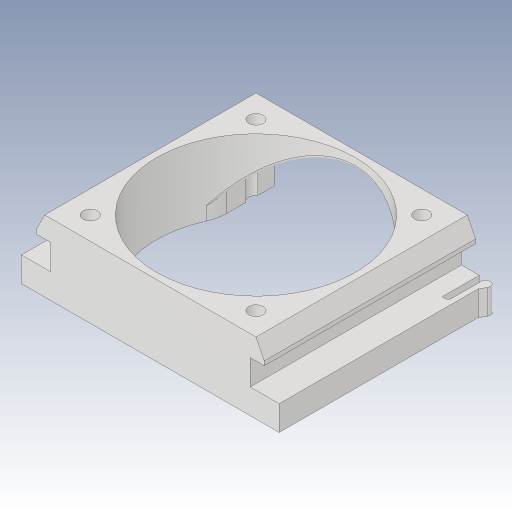
# Autodesk Inventor part: BT016_huenin20_24
Saved by Autodesk Inventor 2023.3 (Build 273359000, 359)
## iProperties
Company: HTBLA Kaindorf
RuleStatus: InUse
Created: 2025-01-29
Part Number: BT016_huenin20_24
Project: Fiberprinter-Hotend
Material: ABS-Kunststoff
Description: Bauteilkühllüfter_befestigung
Document SubType Name: Modeling
Designer: huenin20
Density: 1.06 g/cm^3
Appearance: Glatt - Weiß
Mass: 1.79395 g
Surface Area: 23.0026 cm^2
Volume: 1.69241 cm^3
AfterDocNew0: iProperties-Editor_aufrufen
Author: nicob
Keywords: 2024
Autodesk Inventor part; units mm, degrees
ref_plane "YZ Plane" through (0, 0, 0) normal (1, 0, 0) x (0, 1, 0)
ref_plane "XZ Plane" through (0, 0, 0) normal (0, 1, 0) x (-1, 0, 0)
ref_plane "XY Plane" through (0, 0, 0) normal (0, 0, 1) x (1, 0, 0)
sketch "Skizze3" plane through (0, 0, 0) normal (1, 0, 0) x (0, 1, 0)
  line L0 (0, 0) -> (24.1, 0)
  line L1 (24.1, 0) -> (24.1, -3.075)
  line L2 (24.1, -3.075) -> (27.6, -3.075)
  line L3 (27.6, -3.075) -> (27.6, -6.075)
  line L4 (27.6, -6.075) -> (-3.5, -6.075)
  line L5 (-3.5, -6.075) -> (-3.5, -3.075)
  line L6 (-3.5, -3.075) -> (0, -3.075)
  line L7 (0, -3.075) -> (0, 0)
  line L8 (0, 0) -> (-1.7, 0)
  line L9 (-1.7, 0) -> (-1.7, 2.5)
  line L10 (-1.7, 2.5) -> (25.8, 2.5)
  line L11 (25.8, 2.5) -> (25.8, 0)
  line L12 (25.8, 0) -> (24.1, 0)
  dimension "d4" = 24.1
  dimension "d5" = 3.075
  dimension "d6" = 3
  dimension "d7" = 3.5
  dimension "d15" = 27.5
  dimension "d16" = 2.5
  constraints: 26 end point, 9 perpendicular, 3 collinear, 3 point on line, 2 horizontal, 1 horizontal alignment
  measures "d4" distance of L0.start L0.end
  measures "d5" distance of L0.end L1.end
  measures "d6" distance of L2.end L3.end
  measures "d7" distance of L5.end L6.end
  measures "d15" distance of L9.end L10.end
  measures "d16" distance of L8.end L9.end
extrude "Extrusion3" add sketch "Skizze3" along normal blind 25.5
ref_plane "Arbeitsebene1" through (0, 12.05, -3.075) normal (0, 1, 0) x (1, 0, 0)
sketch "Skizze4" plane through (0, 12.05, -3.075) normal (0, 1, 0) x (1, 0, 0)
  line L0 (0, 3) -> (0, 0) projected
  line L1 (0, 3) -> (25.5, 3) projected
  line L2 (0, -4.5) -> (8.9382, 3)
  line L3 (0, 0) -> (0, -3.075) projected
  line L4 (0, -3.075) -> (0, -5.575) projected
  dimension "d10" = 7.5
  dimension "d14" = 140
  constraints: 2 end point, 2 point on line
  measures "d10" distance of L0.start L2.start
  measures "d14" angle of L1 L2
extrude "Extrusion4" cut sketch "Skizze4" along normal mid plane 21
chamfer "Fase1" distance 1 distance2 2 2 edges at (12.75, -1.7, 2.5) (12.75, 25.8, 2.5) measured on face at (12.75, 25.3, 2.5) measured on face at (12.75, -1.2, 2.5)
sketch "Skizze5" plane through (0, -0.7, 2.5) normal (0, 0, 1) x (1, 0, 0)
  circle A0 centre (12.75, 12.75) radius 12
  line L0 (25.5, 25.5) -> (25.5, 0) projected
  point P0 (0, 0.7)
  point P1 (25.5, 12.75)
  dimension "d20" = 24
  dimension "d21" = 12.75
  constraints: 1 centre point, 1 horizontal alignment, 1 midpoint
  measures "d20" diameter of A0
  measures "d21" distance from line of L0 A0.centre
extrude "Extrusion5" cut sketch "Skizze5" against normal blind 20
fillet "Rundung1" radius 5 2 edges at (6.9405, 1.55, -5.2369) (6.9405, 22.55, -5.2369)
fillet "Rundung2" radius 0.4 3 edges at (7.3765, 1.3204, -4.7646) (0.75, 12.05, 0.7957) (7.3765, 22.7796, -4.7646)
sketch "Skizze6" plane through (0, -0.7, 2.5) normal (0, 0, 1) x (1, 0, 0)
  circle A0 centre (12.75, 12.75) radius 12 projected
  line L0 (2.75, 2.75) -> (22.75, 2.75) construction
  line L1 (22.75, 2.75) -> (22.75, 22.75) construction
  line L2 (22.75, 22.75) -> (2.75, 22.75) construction
  line L3 (2.75, 22.75) -> (2.75, 2.75) construction
  line L4 (2.75, 2.75) -> (22.75, 22.75) construction
  line L5 (22.75, 2.75) -> (2.75, 22.75) construction
  point P0 (0, 0.7)
  point P1 (12.75, 12.75)
  dimension "d29" = 20
  constraints: 12 end point, 4 coincident, 2 midpoint, 2 parallel, 2 perpendicular, 1 horizontal
  measures "d29" distance of L1.end L2.end
hole "Bohrung1" at (22.75, 2.05, 2.5) at (2.75, 2.05, 2.5) at (2.75, 22.05, 2.5) at (22.75, 22.05, 2.5) direction (0, 0, -1) diameter 1.75 end through all
sketch "Skizze7" plane through (25.5, 27.6, -6.075) normal (0, 0, -1) x (-1, 0, 0)
  arc A0 (23.4681, -5.05) -> (22.0319, -5.05) centre (22.75, -5.55) ccw projected
  line L0 (23.4681, -5.05) -> (25.5, -5.05) projected
  line L1 (25.5, -5.05) -> (25.5, 0) projected
  line L2 (25.5, 0) -> (0, 0) projected
  line L3 (0, -31.1) -> (0, 0) projected
  line L4 (25.5, -31.1) -> (0, -31.1) projected
  line L5 (25.5, -31.1) -> (25.5, -26.05) projected
  line L6 (25.5, -26.05) -> (23.4681, -26.05) projected
  arc A1 (22.0319, -26.05) -> (23.4681, -26.05) centre (22.75, -25.55) ccw projected
  line L7 (22.0319, -26.05) -> (19.7321, -26.05) projected
  arc A2 (19.7321, -26.05) -> (17.6786, -26.4912) centre (19.7321, -31.05) ccw projected
  arc A3 (17.6786, -4.6088) -> (17.6786, -26.4912) centre (12.75, -15.55) ccw projected
  arc A4 (17.6786, -4.6088) -> (19.7321, -5.05) centre (19.7321, -0.05) ccw projected
  line L8 (19.7321, -5.05) -> (22.0319, -5.05) projected
  circle A5 centre (2.75, -25.55) radius 0.875 projected
  circle A6 centre (2.75, -5.55) radius 0.875 projected
  line L9 (25.5, 0) -> (0, 0) projected
  line L10 (21, 0) -> (21, -1.35)
  line L11 (21, -1.35) -> (25.5, -1.35)
  line L12 (21, -0.6) -> (25.5, -0.6)
  line L13 (25.5, -5.05) -> (25.5, 0) projected
  circle A7 centre (25, 0) radius 0.5
  point P0 (25.5, -27.6)
  point P1 (24.5, 0)
  dimension "d40" = 1
  dimension "d38" = 1.35
  dimension "d39" = 0.6
  dimension "d41" = 4.5
  constraints: 6 end point, 5 point on line, 1 horizontal, 1 perpendicular, 1 vertical, 3 other
  measures "d38" distance of L10.start L10.end
  measures "d39" distance between parallel lines of L2 L12
  measures "d41" distance of L10.end L11.end
extrude "Extrusion6" cut sketch "Skizze7" against normal up to surface (3 mm away) contours L11 L10 L12 L1
extrude "Extrusion7" add sketch "Skizze7" against normal up to surface (3 mm away) contours L2 A7 picked at (25.0947, 0.1372)
fillet "Rundung3" radius 0.4 2 edges at (0, 27, -4.575) (4.5, 27, -4.575)
ref_plane "Arbeitsebene2" through (0, 12.05, -6.075) normal (0, -1, 0) x (1, 0, 0)
mirror "Spiegeln1" about plane through (0, 12.05, -6.075) normal (0, -1, 0) of "Rundung3", "Extrusion7", "Extrusion6"
chamfer "Fase3" distance 0.5 angle 45 2 edges at (1, 27.6, -4.575) (1, -3.5, -4.575)
